Autodesk Fusion 360 part; units mm, degrees
(part 2 of 2)
sketch "Sketch49" plane through (0, 0, 3) normal (0, 0, 1) x (-1, 0, 0)
  line L0 (139.9, 32) -> (135, 32)
  line L1 (135, 32) -> (135, 34)
  line L2 (135, 34) -> (139.9, 34)
  line L3 (139.9, 34) -> (139.9, 32)
  circle A0 centre (127.45, 30.3) radius 1.5
  circle A1 centre (147.45, 30.3) radius 1.5
  arc A2 (127.45, 32.75) -> (127.45, 27.85) centre (127.45, 30.3) ccw
  line L4 (127.45, 27.85) -> (129.5, 27.85)
  line L5 (129.5, 27.85) -> (129.5, 25)
  line L6 (129.5, 25) -> (145.4, 25)
  line L7 (145.4, 25) -> (145.4, 27.85)
  line L8 (145.4, 27.85) -> (147.45, 27.85)
  arc A3 (147.45, 27.85) -> (147.45, 32.75) centre (147.45, 30.3) ccw
  line L9 (147.45, 32.75) -> (145.4, 32.75)
  line L10 (145.4, 32.75) -> (145.4, 35.6)
  line L11 (145.4, 35.6) -> (129.5, 35.6)
  line L12 (129.5, 35.6) -> (129.5, 32.75)
  line L13 (129.5, 32.75) -> (127.45, 32.75)
  line L14 (130, 25.5) -> (145, 25.5)
  line L15 (145, 25.5) -> (145, 27.5)
  line L16 (145, 27.5) -> (130, 27.5)
  line L17 (130, 27.5) -> (130, 25.5)
  constraint horizontal L14
  constraint vertical L15
  constraint horizontal L16
  constraint vertical L17
extrude "Extrude59" cut sketch "Sketch49" against normal blind 1 contours L14 L15 L16 L17 bodies 7
sketch "Sketch50" plane through (0, 0, 3) normal (0, 0, 1) x (-1, 0, 0)
  circle A0 centre (106.91, 41.51) radius 0.83
  circle A1 centre (106.91, 26.27) radius 0.83
  circle A2 centre (66.27, 41.51) radius 0.83
  circle A3 centre (66.27, 26.27) radius 0.83
  line L0 (65, 39) -> (71, 39)
  line L1 (71, 39) -> (71, 29)
  line L2 (71, 29) -> (65, 29)
  line L3 (65, 29) -> (65, 25)
  line L4 (65, 25) -> (108.18, 25)
  line L5 (108.18, 25) -> (108.18, 42.78)
  line L6 (108.18, 42.78) -> (65, 42.78)
  line L7 (65, 42.78) -> (65, 39)
  line L8 (105, 28) -> (93, 28)
  line L9 (93, 28) -> (93, 40)
  line L10 (93, 40) -> (105, 40)
  line L11 (105, 40) -> (105, 28)
  line L12 (76.4925, 33.236) -> (76.4925, 33)
  line L13 (76.4925, 33) -> (75, 33)
  line L14 (75, 33) -> (75, 35)
  line L15 (75, 35) -> (76.4461, 35)
  line L16 (76.4461, 35) -> (76.4461, 34.764)
  line L17 (76.4461, 34.764) -> (75.2647, 34.764)
  line L18 (75.2647, 34.764) -> (75.2647, 34.1514)
  line L19 (75.2647, 34.1514) -> (76.3711, 34.1514)
  line L20 (76.3711, 34.1514) -> (76.3711, 33.9168)
  line L21 (76.3711, 33.9168) -> (75.2647, 33.9168)
  line L22 (75.2647, 33.9168) -> (75.2647, 33.236)
  line L23 (75.2647, 33.236) -> (76.4925, 33.236)
  spline S0 degree 3 poles (82.4529, 33.369) (82.4332, 33.3474) (82.3952, 33.3057) (82.3642, 33.2587) (82.3493, 33.236) knots 0 0 0 0 0.008766 0.016888 0.016888 0.016888 0.016888
  line L24 (82.3493, 33.236) -> (83.3302, 33.236)
  line L25 (83.3302, 33.236) -> (83.3302, 33)
  line L26 (83.3302, 33) -> (82.0082, 33)
  spline S1 degree 3 poles (82.0082, 33) (82.0087, 33.0292) (82.0097, 33.0875) (82.0278, 33.1429) (82.0368, 33.1705) knots 0 0 0 0 0.008716 0.017379 0.017379 0.017379 0.017379
  spline S2 degree 3 poles (82.0368, 33.1705) (82.057, 33.2163) (82.0991, 33.312) (82.1644, 33.3938) (82.1985, 33.4366) knots 0 0 0 0 0.014925 0.031247 0.031247 0.031247 0.031247
  spline S3 degree 3 poles (82.1985, 33.4366) (82.2429, 33.4845) (82.3431, 33.5927) (82.4566, 33.687) (82.5198, 33.7394) knots 0 0 0 0 0.019599 0.044195 0.044195 0.044195 0.044195
  spline S4 degree 3 poles (82.5198, 33.7394) (82.6137, 33.8164) (82.7719, 33.9461) (82.9059, 34.1003) (82.9604, 34.163) knots 0 0 0 0 0.036337 0.061217 0.061217 0.061217 0.061217
  spline S5 degree 3 poles (82.9604, 34.163) (82.9938, 34.2119) (83.0551, 34.3018) (83.0688, 34.4094) (83.075, 34.4584) knots 0 0 0 0 0.017457 0.032082 0.032082 0.032082 0.032082
  spline S6 degree 3 poles (83.075, 34.4584) (83.0707, 34.5051) (83.0621, 34.5983) (83.0011, 34.6693) (82.9707, 34.7046) knots 0 0 0 0 0.013706 0.027345 0.027345 0.027345 0.027345
  spline S7 degree 3 poles (82.9707, 34.7046) (82.9322, 34.7339) (82.8519, 34.7948) (82.751, 34.8015) (82.6985, 34.8049) knots 0 0 0 0 0.014181 0.029581 0.029581 0.029581 0.029581
  spline S8 degree 3 poles (82.6985, 34.8049) (82.6432, 34.8014) (82.5376, 34.7945) (82.4544, 34.7295) (82.4147, 34.6985) knots 0 0 0 0 0.016182 0.030941 0.030941 0.030941 0.030941
  spline S9 degree 3 poles (82.4147, 34.6985) (82.3837, 34.6579) (82.3174, 34.5712) (82.3106, 34.4619) (82.307, 34.4038) knots 0 0 0 0 0.015007 0.032013 0.032013 0.032013 0.032013
  line L27 (82.307, 34.4038) -> (82.0546, 34.4297)
  spline S10 degree 3 poles (82.0546, 34.4297) (82.0672, 34.5164) (82.0908, 34.6793) (82.199, 34.8025) (82.2497, 34.8602) knots 0 0 0 0 0.025635 0.048167 0.048167 0.048167 0.048167
  spline S11 degree 3 poles (82.2497, 34.8602) (82.3136, 34.9033) (82.4505, 34.9955) (82.6159, 35.0038) (82.704, 35.0082) knots 0 0 0 0 0.022714 0.048594 0.048594 0.048594 0.048594
  spline S12 degree 3 poles (82.704, 35.0082) (82.793, 35.0033) (82.9609, 34.9941) (83.0961, 34.8951) (83.1596, 34.8486) knots 0 0 0 0 0.026091 0.049213 0.049213 0.049213 0.049213
  spline S13 degree 3 poles (83.1596, 34.8486) (83.2086, 34.792) (83.307, 34.6782) (83.3206, 34.5283) (83.3274, 34.4529) knots 0 0 0 0 0.021858 0.043952 0.043952 0.043952 0.043952
  spline S14 degree 3 poles (83.3274, 34.4529) (83.3253, 34.4129) (83.3209, 34.3317) (83.2926, 34.2555) (83.2783, 34.2169) knots 0 0 0 0 0.011966 0.024231 0.024231 0.024231 0.024231
  spline S15 degree 3 poles (83.2783, 34.2169) (83.2579, 34.1763) (83.2137, 34.0882) (83.1498, 34.0132) (83.1153, 33.9727) knots 0 0 0 0 0.013577 0.029457 0.029457 0.029457 0.029457
  spline S16 degree 3 poles (83.1153, 33.9727) (83.0654, 33.9213) (82.9453, 33.7975) (82.8137, 33.686) (82.7367, 33.6207) knots 0 0 0 0 0.021476 0.051719 0.051719 0.051719 0.051719
  spline S17 degree 3 poles (82.7367, 33.6207) (82.6755, 33.5697) (82.5783, 33.4886) (82.4868, 33.4013) (82.4529, 33.369) knots 0 0 0 0 0.023909 0.03794 0.03794 0.03794 0.03794
  spline S18 degree 3 poles (81.1228, 32.9645) (81.0397, 32.9702) (80.8789, 32.9811) (80.7486, 33.0757) (80.6855, 33.1214) knots 0 0 0 0 0.024413 0.047298 0.047298 0.047298 0.047298
  spline S19 degree 3 poles (80.6855, 33.1214) (80.6337, 33.1783) (80.5281, 33.2944) (80.5009, 33.4491) (80.487, 33.528) knots 0 0 0 0 0.022603 0.04608 0.04608 0.04608 0.04608
  line L28 (80.487, 33.528) -> (80.7326, 33.5607)
  spline S20 degree 3 poles (80.7326, 33.5607) (80.7468, 33.4984) (80.7721, 33.3868) (80.8445, 33.2988) (80.8765, 33.2599) knots 0 0 0 0 0.018844 0.033755 0.033755 0.033755 0.033755
  spline S21 degree 3 poles (80.8765, 33.2599) (80.9127, 33.233) (80.9862, 33.1784) (81.0776, 33.1714) (81.1241, 33.1678) knots 0 0 0 0 0.01322 0.026904 0.026904 0.026904 0.026904
  spline S22 degree 3 poles (81.1241, 33.1678) (81.1795, 33.1727) (81.2896, 33.1824) (81.3746, 33.2528) (81.4168, 33.2879) knots 0 0 0 0 0.016258 0.032307 0.032307 0.032307 0.032307
  spline S23 degree 3 poles (81.4168, 33.2879) (81.4516, 33.3306) (81.5221, 33.4173) (81.5314, 33.5288) (81.5362, 33.5853) knots 0 0 0 0 0.016147 0.032721 0.032721 0.032721 0.032721
  spline S24 degree 3 poles (81.5362, 33.5853) (81.532, 33.6387) (81.5239, 33.7433) (81.4579, 33.8246) (81.4256, 33.8643) knots 0 0 0 0 0.015678 0.030648 0.030648 0.030648 0.030648
  spline S25 degree 3 poles (81.4256, 33.8643) (81.3856, 33.8963) (81.3035, 33.962) (81.1985, 33.97) (81.1446, 33.9741) knots 0 0 0 0 0.015013 0.030806 0.030806 0.030806 0.030806
  spline S26 degree 3 poles (81.1446, 33.9741) (81.1185, 33.9725) (81.0599, 33.969) (81.0029, 33.9547) (80.9714, 33.9468) knots 0 0 0 0 0.00784 0.017573 0.017573 0.017573 0.017573
  line L29 (80.9714, 33.9468) -> (80.9986, 34.1623)
  spline S27 degree 3 poles (80.9986, 34.1623) (81.006, 34.1616) (81.0192, 34.1601) (81.0324, 34.1598) (81.0382, 34.1596) knots 0 0 0 0 0.002226 0.003967 0.003967 0.003967 0.003967
  spline S28 degree 3 poles (81.0382, 34.1596) (81.0889, 34.1629) (81.1892, 34.1693) (81.2771, 34.2176) (81.3206, 34.2415) knots 0 0 0 0 0.015044 0.029725 0.029725 0.029725 0.029725
  spline S29 degree 3 poles (81.3206, 34.2415) (81.3572, 34.2735) (81.4333, 34.3401) (81.4417, 34.4413) (81.4461, 34.4939) knots 0 0 0 0 0.014029 0.029194 0.029194 0.029194 0.029194
  spline S30 degree 3 poles (81.4461, 34.4939) (81.4426, 34.5367) (81.4356, 34.621) (81.3814, 34.6857) (81.3547, 34.7176) knots 0 0 0 0 0.012556 0.024703 0.024703 0.024703 0.024703
  spline S31 degree 3 poles (81.3547, 34.7176) (81.3212, 34.7435) (81.2518, 34.7971) (81.1641, 34.8031) (81.1187, 34.8063) knots 0 0 0 0 0.012404 0.025721 0.025721 0.025721 0.025721
  spline S32 degree 3 poles (81.1187, 34.8063) (81.0733, 34.8029) (80.9848, 34.7963) (80.9143, 34.7425) (80.8799, 34.7162) knots 0 0 0 0 0.013323 0.026012 0.026012 0.026012 0.026012
  spline S33 degree 3 poles (80.8799, 34.7162) (80.8507, 34.6802) (80.7864, 34.6012) (80.7675, 34.5007) (80.7572, 34.4461) knots 0 0 0 0 0.013719 0.030088 0.030088 0.030088 0.030088
  line L30 (80.7572, 34.4461) -> (80.5116, 34.4898)
  spline S34 degree 3 poles (80.5116, 34.4898) (80.53, 34.5662) (80.565, 34.7119) (80.6675, 34.8207) (80.7162, 34.8724) knots 0 0 0 0 0.023119 0.04407 0.04407 0.04407 0.04407
  spline S35 degree 3 poles (80.7162, 34.8724) (80.774, 34.912) (80.8935, 34.994) (81.0383, 35.0033) (81.1132, 35.0082) knots 0 0 0 0 0.020598 0.042654 0.042654 0.042654 0.042654
  spline S36 degree 3 poles (81.1132, 35.0082) (81.1664, 35.0054) (81.2711, 35) (81.3673, 34.9584) (81.4147, 34.9379) knots 0 0 0 0 0.015821 0.03118 0.03118 0.03118 0.03118
  spline S37 degree 3 poles (81.4147, 34.9379) (81.4577, 34.9129) (81.5416, 34.8639) (81.598, 34.7848) (81.6255, 34.7462) knots 0 0 0 0 0.014725 0.02878 0.02878 0.02878 0.02878
  spline S38 degree 3 poles (81.6255, 34.7462) (81.6468, 34.7054) (81.689, 34.6245) (81.6953, 34.5335) (81.6985, 34.4884) knots 0 0 0 0 0.013662 0.027054 0.027054 0.027054 0.027054
  spline S39 degree 3 poles (81.6985, 34.4884) (81.6957, 34.4463) (81.69, 34.3624) (81.6492, 34.2889) (81.6289, 34.2524) knots 0 0 0 0 0.012502 0.024877 0.024877 0.024877 0.024877
  spline S40 degree 3 poles (81.6289, 34.2524) (81.602, 34.2183) (81.5457, 34.147) (81.465, 34.1051) (81.4229, 34.0832) knots 0 0 0 0 0.012871 0.026927 0.026927 0.026927 0.026927
  spline S41 degree 3 poles (81.4229, 34.0832) (81.4782, 34.0666) (81.5853, 34.0345) (81.6616, 33.9529) (81.6985, 33.9134) knots 0 0 0 0 0.016967 0.032892 0.032892 0.032892 0.032892
  spline S42 degree 3 poles (81.6985, 33.9134) (81.7271, 33.8663) (81.7873, 33.7673) (81.7935, 33.6514) (81.7967, 33.5907) knots 0 0 0 0 0.016275 0.034196 0.034196 0.034196 0.034196
  spline S43 degree 3 poles (81.7967, 33.5907) (81.7887, 33.5067) (81.7726, 33.3382) (81.6614, 33.2106) (81.6057, 33.1467) knots 0 0 0 0 0.024665 0.049435 0.049435 0.049435 0.049435
  spline S44 degree 3 poles (81.6057, 33.1467) (81.5366, 33.0935) (81.3942, 32.9843) (81.2149, 32.9712) (81.1228, 32.9645) knots 0 0 0 0 0.025577 0.052634 0.052634 0.052634 0.052634
  line L31 (78.9864, 33.8131) -> (78.9864, 33)
  line L32 (78.9864, 33) -> (78.7217, 33)
  line L33 (78.7217, 33) -> (78.7217, 35)
  line L34 (78.7217, 35) -> (79.4761, 35)
  spline S45 degree 3 poles (79.4761, 35) (79.5348, 34.9998) (79.6366, 34.9995) (79.7375, 34.9864) (79.7804, 34.9809) knots 0 0 0 0 0.017571 0.030509 0.030509 0.030509 0.030509
  spline S46 degree 3 poles (79.7804, 34.9809) (79.8265, 34.9715) (79.9139, 34.9538) (79.9909, 34.9088) (80.0273, 34.8874) knots 0 0 0 0 0.014001 0.026563 0.026563 0.026563 0.026563
  spline S47 degree 3 poles (80.0273, 34.8874) (80.0592, 34.8615) (80.1253, 34.8078) (80.1663, 34.7331) (80.1876, 34.6944) knots 0 0 0 0 0.012214 0.025303 0.025303 0.025303 0.025303
  spline S48 degree 3 poles (80.1876, 34.6944) (80.2053, 34.6515) (80.2414, 34.5642) (80.246, 34.4697) (80.2483, 34.4216) knots 0 0 0 0 0.013801 0.028138 0.028138 0.028138 0.028138
  spline S49 degree 3 poles (80.2483, 34.4216) (80.242, 34.3403) (80.2296, 34.1805) (80.1333, 34.0526) (80.0859, 33.9898) knots 0 0 0 0 0.023898 0.046996 0.046996 0.046996 0.046996
  spline S50 degree 3 poles (80.0859, 33.9898) (80.0124, 33.9386) (79.8379, 33.8171) (79.6234, 33.8146) (79.4993, 33.8131) knots 0 0 0 0 0.026356 0.062507 0.062507 0.062507 0.062507
  line L35 (79.4993, 33.8131) -> (78.9864, 33.8131)
  spline S51 degree 3 poles (77.1658, 33.045) (77.1081, 33.0744) (76.9944, 33.1323) (76.9164, 33.2333) (76.8779, 33.2831) knots 0 0 0 0 0.019136 0.037772 0.037772 0.037772 0.037772
  spline S52 degree 3 poles (76.8779, 33.2831) (76.8472, 33.3383) (76.785, 33.4502) (76.7738, 33.5778) (76.7681, 33.6426) knots 0 0 0 0 0.018713 0.037965 0.037965 0.037965 0.037965
  line L36 (76.7681, 33.6426) -> (77.0177, 33.6644)
  spline S53 degree 3 poles (77.0177, 33.6644) (77.0248, 33.6179) (77.038, 33.5309) (77.0805, 33.454) (77.1003, 33.4181) knots 0 0 0 0 0.013975 0.026155 0.026155 0.026155 0.026155
  spline S54 degree 3 poles (77.1003, 33.4181) (77.1262, 33.3871) (77.1817, 33.3205) (77.2598, 33.2827) (77.3015, 33.2626) knots 0 0 0 0 0.012002 0.025694 0.025694 0.025694 0.025694
  spline S55 degree 3 poles (77.3015, 33.2626) (77.3493, 33.2453) (77.4485, 33.2094) (77.5539, 33.2054) (77.6085, 33.2033) knots 0 0 0 0 0.015163 0.031432 0.031432 0.031432 0.031432
  spline S56 degree 3 poles (77.6085, 33.2033) (77.6564, 33.2047) (77.7476, 33.2075) (77.8346, 33.2352) (77.8759, 33.2483) knots 0 0 0 0 0.014301 0.027232 0.027232 0.027232 0.027232
  spline S57 degree 3 poles (77.8759, 33.2483) (77.9113, 33.2637) (77.9778, 33.2926) (78.0259, 33.3466) (78.0484, 33.3718) knots 0 0 0 0 0.011435 0.021444 0.021444 0.021444 0.021444
  spline S58 degree 3 poles (78.0484, 33.3718) (78.0649, 33.3983) (78.0976, 33.4509) (78.1026, 33.5125) (78.105, 33.543) knots 0 0 0 0 0.009237 0.018267 0.018267 0.018267 0.018267
  spline S59 degree 3 poles (78.105, 33.543) (78.1029, 33.5732) (78.0987, 33.6327) (78.0664, 33.6827) (78.0505, 33.7074) knots 0 0 0 0 0.008921 0.017573 0.017573 0.017573 0.017573
  spline S60 degree 3 poles (78.0505, 33.7074) (78.0275, 33.7305) (77.9759, 33.7824) (77.908, 33.8101) (77.8704, 33.8254) knots 0 0 0 0 0.009698 0.021725 0.021725 0.021725 0.021725
  spline S61 degree 3 poles (77.8704, 33.8254) (77.8274, 33.8392) (77.7102, 33.8767) (77.5903, 33.905) (77.5143, 33.9229) knots 0 0 0 0 0.013533 0.036931 0.036931 0.036931 0.036931
  spline S62 degree 3 poles (77.5143, 33.9229) (77.4354, 33.9418) (77.3033, 33.9733) (77.1784, 34.0264) (77.1282, 34.0477) knots 0 0 0 0 0.024297 0.040637 0.040637 0.040637 0.040637
  spline S63 degree 3 poles (77.1282, 34.0477) (77.0843, 34.0732) (77.0008, 34.1214) (76.9424, 34.1978) (76.9147, 34.234) knots 0 0 0 0 0.015064 0.02858 0.02858 0.02858 0.02858
  spline S64 degree 3 poles (76.9147, 34.234) (76.8942, 34.2724) (76.8527, 34.3503) (76.8473, 34.4384) (76.8445, 34.4829) knots 0 0 0 0 0.012908 0.026139 0.026139 0.026139 0.026139
  spline S65 degree 3 poles (76.8445, 34.4829) (76.8482, 34.5328) (76.8557, 34.6336) (76.9054, 34.7216) (76.9304, 34.766) knots 0 0 0 0 0.014805 0.02991 0.02991 0.02991 0.02991
  spline S66 degree 3 poles (76.9304, 34.766) (76.9633, 34.8076) (77.0312, 34.8938) (77.1302, 34.9413) (77.1814, 34.9659) knots 0 0 0 0 0.01568 0.032466 0.032466 0.032466 0.032466
  spline S67 degree 3 poles (77.1814, 34.9659) (77.239, 34.9858) (77.3579, 35.0269) (77.4836, 35.0316) (77.5484, 35.0341) knots 0 0 0 0 0.018164 0.037509 0.037509 0.037509 0.037509
  spline S68 degree 3 poles (77.5484, 35.0341) (77.6189, 35.0317) (77.7532, 35.0272) (77.8802, 34.9834) (77.9407, 34.9625) knots 0 0 0 0 0.021001 0.040071 0.040071 0.040071 0.040071
  spline S69 degree 3 poles (77.9407, 34.9625) (77.9936, 34.9365) (78.0966, 34.8858) (78.1674, 34.7956) (78.2019, 34.7517) knots 0 0 0 0 0.017437 0.033952 0.033952 0.033952 0.033952
  spline S70 degree 3 poles (78.2019, 34.7517) (78.2289, 34.7034) (78.2836, 34.6052) (78.2946, 34.4933) (78.3001, 34.4366) knots 0 0 0 0 0.016416 0.033327 0.033327 0.033327 0.033327
  line L37 (78.3001, 34.4366) -> (78.0464, 34.4175)
  spline S71 degree 3 poles (78.0464, 34.4175) (78.0368, 34.4756) (78.0189, 34.5852) (77.9433, 34.666) (77.9079, 34.704) knots 0 0 0 0 0.017238 0.032462 0.032462 0.032462 0.032462
  spline S72 degree 3 poles (77.9079, 34.704) (77.8604, 34.7321) (77.7535, 34.7955) (77.6287, 34.7989) (77.5593, 34.8008) knots 0 0 0 0 0.016321 0.036707 0.036707 0.036707 0.036707
  spline S73 degree 3 poles (77.5593, 34.8008) (77.4884, 34.7997) (77.3642, 34.7979) (77.2559, 34.7384) (77.2094, 34.7128) knots 0 0 0 0 0.02087 0.036564 0.036564 0.036564 0.036564
  spline S74 degree 3 poles (77.2094, 34.7128) (77.1774, 34.6828) (77.1156, 34.6248) (77.1048, 34.5411) (77.0996, 34.5007) knots 0 0 0 0 0.012728 0.024562 0.024562 0.024562 0.024562
  spline S75 degree 3 poles (77.0996, 34.5007) (77.1027, 34.4665) (77.1089, 34.3986) (77.1547, 34.3483) (77.1774, 34.3233) knots 0 0 0 0 0.010013 0.019843 0.019843 0.019843 0.019843
  spline S76 degree 3 poles (77.1774, 34.3233) (77.2227, 34.2981) (77.3472, 34.2287) (77.4873, 34.1994) (77.5764, 34.1808) knots 0 0 0 0 0.01549 0.042576 0.042576 0.042576 0.042576
  spline S77 degree 3 poles (77.5764, 34.1808) (77.6678, 34.1603) (77.818, 34.1268) (77.9625, 34.0739) (78.0191, 34.0532) knots 0 0 0 0 0.028046 0.046113 0.046113 0.046113 0.046113
  spline S78 degree 3 poles (78.0191, 34.0532) (78.0724, 34.0262) (78.1723, 33.9754) (78.2437, 33.8894) (78.2769, 33.8493) knots 0 0 0 0 0.017708 0.033187 0.033187 0.033187 0.033187
  spline S79 degree 3 poles (78.2769, 33.8493) (78.3012, 33.806) (78.3508, 33.7176) (78.357, 33.6165) (78.3602, 33.5648) knots 0 0 0 0 0.014678 0.02998 0.02998 0.02998 0.02998
  spline S80 degree 3 poles (78.3602, 33.5648) (78.3561, 33.512) (78.348, 33.405) (78.2954, 33.3114) (78.2688, 33.264) knots 0 0 0 0 0.015669 0.031781 0.031781 0.031781 0.031781
  spline S81 degree 3 poles (78.2688, 33.264) (78.2342, 33.2192) (78.1628, 33.1268) (78.0594, 33.0724) (78.0061, 33.0443) knots 0 0 0 0 0.016779 0.034595 0.034595 0.034595 0.034595
  spline S82 degree 3 poles (78.0061, 33.0443) (77.9462, 33.0215) (77.8221, 32.9741) (77.6893, 32.9687) (77.6207, 32.9659) knots 0 0 0 0 0.019123 0.039562 0.039562 0.039562 0.039562
  spline S83 degree 3 poles (77.6207, 32.9659) (77.5368, 32.968) (77.381, 32.972) (77.2337, 33.022) (77.1658, 33.045) knots 0 0 0 0 0.025027 0.046416 0.046416 0.046416 0.046416
  line L38 (68, 25) -> (105, 25)
  line L39 (105, 25) -> (105, 27)
  line L40 (105, 27) -> (68, 27)
  line L41 (68, 27) -> (68, 25)
  line L42 (68, 41) -> (68, 42.78)
  line L43 (68, 42.78) -> (105, 42.78)
  line L44 (105, 42.78) -> (105, 40.78)
  line L45 (105, 40.78) -> (68, 40.78)
  line L46 (68, 40.78) -> (68, 42.78)
  dimension "d258" = 2
  constraint horizontal L38
  constraint vertical L39
  constraint horizontal L40
  constraint vertical L41
  constraint coincident L4 L38.start
  constraint coincident L6 L42.end
  constraint perpendicular L6 L42
  constraint horizontal L43
  constraint vertical L44
  constraint horizontal L45
  constraint vertical L46
  measures "d258" distance of L42.end L45.end
extrude "Extrude60" cut sketch "Sketch50" against normal blind 1 contours L6 L42 L43 L44 L45 L46 | L4 L38 L39 L40 L41 bodies 4
sketch "Sketch51" plane through (0, 0, 2) normal (0, 0, 1) x (-1, 0, 0)
  line L0 (68, 27) -> (68, 25)
  line L1 (68, 25) -> (105, 25)
  line L2 (105, 25) -> (105, 27)
  line L3 (105, 27) -> (68, 27)
sketch "Sketch52" plane through (0, 0, 3) normal (0, 0, 1) x (-1, 0, 0)
  line L0 (145, 25.5) -> (130, 25.5)
  line L1 (130, 25.5) -> (130, 27.5)
  line L2 (130, 27.5) -> (145, 27.5)
  line L3 (145, 27.5) -> (145, 25.5)
  line L4 (139.9, 32) -> (135, 32)
  line L5 (135, 32) -> (135, 34)
  line L6 (135, 34) -> (139.9, 34)
  line L7 (139.9, 34) -> (139.9, 32)
  circle A0 centre (127.45, 30.3) radius 1.5
  circle A1 centre (147.45, 30.3) radius 1.5
  arc A2 (127.45, 32.75) -> (127.45, 27.85) centre (127.45, 30.3) ccw
  line L8 (127.45, 27.85) -> (129.5, 27.85)
  line L9 (129.5, 27.85) -> (129.5, 25)
  line L10 (129.5, 25) -> (145.4, 25)
  line L11 (145.4, 25) -> (145.4, 27.85)
  line L12 (145.4, 27.85) -> (147.45, 27.85)
  arc A3 (147.45, 27.85) -> (147.45, 32.75) centre (147.45, 30.3) ccw
  line L13 (147.45, 32.75) -> (145.4, 32.75)
  line L14 (145.4, 32.75) -> (145.4, 35.6)
  line L15 (145.4, 35.6) -> (129.5, 35.6)
  line L16 (129.5, 35.6) -> (129.5, 32.75)
  line L17 (129.5, 32.75) -> (127.45, 32.75)
  line L18 (135.0059, 30.3197) -> (139.9059, 30.3369) construction
  line L19 (139.9059, 30.3369) -> (139.9, 32.0172) construction
  line L20 (139.9, 32.0172) -> (135, 32) construction
  line L21 (135, 32) -> (135.0059, 30.3197) construction
  dimension "d265" = 2
  text T0 "ToF" font "Arial" height 2 align centre top in box 4.9 x 1.6803 at (135.0059, 30.3197) x (0.999994, 0.003504) y (-0.003504, 0.999994) spacing 1 kerned
  constraint coincident L4.end
extrude "Extrude61" cut sketch "Sketch52" against normal blind 1 text T0 bodies 7
copy_body "CopyPasteBodies1" bodies 7 makes body 8
move_body "Move2" bodies 8 to x (1, 0, 0) y (0, 1, 0) z (0, 0, 1) at (0.0526, -14.9999, 0)
sketch "Sketch53" plane through (0, 0, 0) normal (0, 0, 1) x (1, 0, 0)
  line L0 (0, -95) -> (-20, -95)
  line L1 (-20, -95) -> (-20, -112.8)
  line L2 (-20, -112.8) -> (0, -112.8)
  line L3 (0, -112.8) -> (0, -95)
  line L4 (-20, -112.8) -> (-7, -112.8)
  line L5 (-7, -112.8) -> (-7, -117.5)
  line L6 (-7, -117.5) -> (-20, -117.5)
  line L7 (-20, -117.5) -> (-20, -112.8)
  line L8 (0, -110) -> (3.8, -110)
  line L9 (3.8, -110) -> (3.8, -109)
  line L10 (3.8, -109) -> (0, -109)
  line L11 (0, -109) -> (0, -110)
  line L12 (-20, -110) -> (-23.8, -110)
  line L13 (-23.8, -110) -> (-23.8, -109)
  line L14 (-23.8, -109) -> (-20, -109)
  line L15 (-20, -109) -> (-20, -110)
  dimension "d269" = 20
  dimension "d270" = 17.8
  dimension "d271" = 4.7
  dimension "d272" = 3.8
  dimension "d273" = 1
  dimension "d274" = 3.8
  constraint horizontal L0
  constraint vertical L1
  constraint horizontal L2
  constraint vertical L3
  constraint horizontal L4
  constraint vertical L5
  constraint horizontal L6
  constraint vertical L7
  constraint horizontal L8
  constraint vertical L9
  constraint horizontal L10
  constraint vertical L11
  constraint coincident L3 L8.start
  constraint horizontal L12
  constraint vertical L13
  constraint horizontal L14
  constraint vertical L15
  constraint coincident L1 L12.start
  measures "d269" distance of L0.start L0.end
  measures "d270" distance of L0.start L2.end
  measures "d271" distance of L1.end L6.end
  measures "d272" distance of L8.start L8.end
  measures "d273" distance of L8.start L10.end
  measures "d274" distance of L12.start L12.end
extrude "Extrude62" add sketch "Sketch53" along normal blind 8 separate body makes body 9
sketch "Sketch54" plane through (0, -117.5, 0) normal (0, -1, 0) x (1, 0, 0)
  line L0 (-20, 0) -> (-7, 0)
  line L1 (-7, 0) -> (-7, 8)
  line L2 (-7, 8) -> (-20, 8)
  line L3 (-20, 8) -> (-20, 0)
  circle A0 centre (-16, 4) radius 3.75
  dimension "d277" = 7.5
  measures "d277" diameter of A0
extrude "Extrude63" cut sketch "Sketch54" against normal blind 2 bodies 9
sketch "Sketch55" plane through (0, -115.5, 0) normal (0, -1, 0) x (1, 0, 0)
  circle A0 centre (-16, 4) radius 3.75
  line L0 (-20, 8) -> (-20, 0)
  line L1 (-20, 0) -> (-7, 0)
  line L2 (-7, 0) -> (-7, 8)
  line L3 (-7, 8) -> (-20, 8)
  line L4 (-16, 8) -> (-7.7253, 5.6358)
  line L5 (-16, 0) -> (-7.7253, 2.3642)
  line L6 (-7, 3.3257) -> (-7, 4.6743)
  arc A1 (-7.7253, 2.3642) -> (-7, 3.3257) centre (-8, 3.3257) ccw
  arc A2 (-7, 4.6743) -> (-7.7253, 5.6358) centre (-8, 4.6743) ccw
  dimension "d280" = 1
  constraint coincident L3 L4.start
  constraint coincident L1 L5.start
  constraint tangent L6 A1
  constraint tangent L5 A1
  constraint tangent L4 A2
  constraint tangent L6 A2
  constraint equal A1 A2
  measures "d280" radius of A1
extrude "Extrude64" cut sketch "Sketch55" against normal blind 2.7 contours L2 L3 L4 A2 | L1 L2 L5 A1 bodies 9
extrude "Extrude65" add 1 faces at (-128, 20.0864, 4.8227) along direction (-1, 0, 0) blind 1 on bodies 6 bodies 6
sketch "Sketch56" plane through (0, 0, 0) normal (0, 0, 1) x (1, 0, 0)
  line L0 (-35, -95) -> (-52.1, -95)
  line L1 (-52.1, -95) -> (-52.1, -116.6)
  line L2 (-52.1, -116.6) -> (-35, -116.6)
  line L3 (-35, -116.6) -> (-35, -95)
  dimension "d285" = 17.1
  dimension "d286" = 21.6
  constraint horizontal L0
  constraint vertical L1
  constraint horizontal L2
  constraint vertical L3
  measures "d285" distance of L0.start L0.end
  measures "d286" distance of L0.start L2.end
extrude "Extrude66" add sketch "Sketch56" along normal blind 3 separate body makes body 10
sketch "Sketch57" plane through (0, 0, 3) normal (0, 0, 1) x (-1, 0, 0)
  line L0 (35, 116.6) -> (35, 95)
  line L1 (35, 95) -> (52.1, 95)
  line L2 (52.1, 95) -> (52.1, 116.6)
  line L3 (52.1, 116.6) -> (35, 116.6)
  circle A0 centre (49.5, 114) radius 2
  dimension "d289" = 4
  measures "d289" diameter of A0
extrude "Extrude67" cut sketch "Sketch57" against normal blind 4.5 contours A0 bodies 10
sketch "Sketch58" plane through (0, 0, 3) normal (0, 0, 1) x (-1, 0, 0)
  circle A0 centre (49.5, 114) radius 2
  line L0 (35, 116.6) -> (35, 95)
  line L1 (35, 95) -> (52.1, 95)
  line L2 (52.1, 95) -> (52.1, 116.6)
  line L3 (52.1, 116.6) -> (35, 116.6)
  line L4 (37, 116) -> (35, 116)
  line L5 (35, 116) -> (35, 96)
  line L6 (35, 96) -> (37, 96)
  line L7 (37, 96) -> (37, 116)
  constraint horizontal L4
  constraint vertical L5
  constraint horizontal L6
  constraint vertical L7
  constraint coincident L0 L5.end
extrude "Extrude68" cut sketch "Sketch58" against normal blind 1 contours L0 L4 L5 L6 L7 bodies 10
sketch "Sketch59" plane through (0, 0, 3) normal (0, 0, 1) x (-1, 0, 0)
  line L0 (37, 96) -> (35, 96)
  line L1 (35, 96) -> (35, 95)
  line L2 (35, 95) -> (52.1, 95)
  line L3 (52.1, 95) -> (52.1, 116.6)
  line L4 (52.1, 116.6) -> (35, 116.6)
  line L5 (35, 116.6) -> (35, 116)
  line L6 (35, 116) -> (37, 116)
  line L7 (37, 116) -> (37, 96)
  circle A0 centre (49.5, 114) radius 2
  line L8 (45, 110) -> (48, 110)
  line L9 (48, 110) -> (48, 107)
  line L10 (48, 107) -> (45, 107)
  line L11 (45, 107) -> (45, 110)
  line L12 (45, 105) -> (47, 105)
  line L13 (47, 105) -> (47, 103)
  line L14 (47, 103) -> (45, 103)
  line L15 (45, 103) -> (45, 105)
  line L16 (39, 113) -> (41, 113)
  line L17 (41, 113) -> (41, 112)
  line L18 (41, 112) -> (39, 112)
  line L19 (39, 112) -> (39, 113)
  constraint horizontal L8
  constraint vertical L9
  constraint horizontal L10
  constraint vertical L11
  constraint horizontal L12
  constraint vertical L13
  constraint horizontal L14
  constraint vertical L15
  constraint horizontal L16
  constraint vertical L17
  constraint horizontal L18
  constraint vertical L19
extrude "Extrude69" add sketch "Sketch59" along normal blind 1 contours L8 L9 L10 L11 | L12 L13 L14 L15 | L16 L17 L18 L19 bodies 10
sketch "Sketch60" plane through (0, 0, 3) normal (0, 0, 1) x (-1, 0, 0)
  line L0 (45, 103) -> (45, 105)
  line L1 (45, 105) -> (47, 105)
  line L2 (47, 105) -> (47, 103)
  line L3 (47, 103) -> (45, 103)
  line L4 (45, 107) -> (45, 110)
  line L5 (45, 110) -> (48, 110)
  line L6 (48, 110) -> (48, 107)
  line L7 (48, 107) -> (45, 107)
  line L8 (39, 112) -> (39, 113)
  line L9 (39, 113) -> (41, 113)
  line L10 (41, 113) -> (41, 112)
  line L11 (41, 112) -> (39, 112)
  line L12 (37, 96) -> (35, 96)
  line L13 (35, 96) -> (35, 95)
  line L14 (35, 95) -> (52.1, 95)
  line L15 (52.1, 95) -> (52.1, 116.6)
  line L16 (52.1, 116.6) -> (35, 116.6)
  line L17 (35, 116.6) -> (35, 116)
  line L18 (35, 116) -> (37, 116)
  line L19 (37, 116) -> (37, 96)
  circle A0 centre (49.5, 114) radius 2
  line L20 (37, 97.7) -> (52.1, 97.7) construction
  line L21 (52.1, 97.7) -> (52.1, 101) construction
  line L22 (52.1, 101) -> (37, 101) construction
  line L23 (37, 101) -> (37, 97.7) construction
  dimension "d296" = 2
  text T0 "IMU" font "Arial" height 2 align centre top in box 15.1 x 3.3 at (37, 97.7) x (1, 0) y (0, 1) spacing 1 kerned
  constraint coincident L15
  constraint coincident L19
extrude "Extrude70" cut sketch "Sketch60" against normal blind 1 text T0 bodies 10
sketch "Sketch61" plane through (0, 0, 0) normal (0, 0, 1) x (1, 0, 0)
  line L0 (-70, -95) -> (-80, -95)
  line L1 (-80, -95) -> (-80, -113)
  line L2 (-80, -113) -> (-70, -113)
  line L3 (-70, -113) -> (-70, -95)
  dimension "d300" = 10
  dimension "d301" = 18
  constraint horizontal L0
  constraint vertical L1
  constraint horizontal L2
  constraint vertical L3
  measures "d300" distance of L0.start L0.end
  measures "d301" distance of L0.start L2.end
extrude "Extrude71" add sketch "Sketch61" along normal blind 3 separate body makes body 11
sketch "Sketch62" plane through (0, 0, 3) normal (0, 0, 1) x (-1, 0, 0)
  line L0 (70, 113) -> (70, 95)
  line L1 (70, 95) -> (80, 95)
  line L2 (80, 95) -> (80, 113)
  line L3 (80, 113) -> (70, 113)
  line L4 (71, 113) -> (79, 113)
  line L5 (79, 113) -> (79, 111)
  line L6 (79, 111) -> (71, 111)
  line L7 (71, 111) -> (71, 113)
  circle A0 centre (73, 98) radius 2.2361
  line L8 (76, 101) -> (79, 101)
  line L9 (79, 101) -> (79, 97)
  line L10 (79, 97) -> (76, 97)
  line L11 (76, 97) -> (76, 101)
  constraint horizontal L4
  constraint vertical L5
  constraint horizontal L6
  constraint vertical L7
  constraint coincident L3 L4.start
  constraint horizontal L8
  constraint vertical L9
  constraint horizontal L10
  constraint vertical L11
extrude "Extrude72" add sketch "Sketch62" along normal blind 2 contours L3 L4 L5 L6 L7 | A0 | L8 L9 L10 L11 bodies 11
sketch "Sketch63" plane through (0, -113, 0) normal (0, -1, 0) x (1, 0, 0)
  line L0 (-80, 0) -> (-70, 0)
  line L1 (-70, 0) -> (-70, 3)
  line L2 (-70, 3) -> (-71, 3)
  line L3 (-71, 3) -> (-71, 5)
  line L4 (-71, 5) -> (-79, 5)
  line L5 (-79, 5) -> (-79, 3)
  line L6 (-79, 3) -> (-80, 3)
  line L7 (-80, 3) -> (-80, 0)
  circle A0 centre (-77.5, 4) radius 0.5385
  circle A1 centre (-72.5, 4) radius 0.5099
  circle A2 centre (-75, 4) radius 0.5
extrude "Extrude73" add sketch "Sketch63" along normal blind 6 contours A0 | A1 | A2 bodies 11
sketch "Sketch64" plane through (0, 0, 3) normal (0, 0, 1) x (-1, 0, 0)
  line L0 (76, 97) -> (76, 101)
  line L1 (76, 101) -> (79, 101)
  line L2 (79, 101) -> (79, 97)
  line L3 (79, 97) -> (76, 97)
  circle A0 centre (73, 98) radius 2.2361
  line L4 (79, 113) -> (79, 111)
  line L5 (79, 111) -> (71, 111)
  line L6 (71, 111) -> (71, 113)
  line L7 (71, 113) -> (70, 113)
  line L8 (70, 113) -> (70, 95)
  line L9 (70, 95) -> (80, 95)
  line L10 (80, 95) -> (80, 113)
  line L11 (80, 113) -> (79, 113)
  line L12 (71, 108) -> (79, 108) construction
  line L13 (79, 108) -> (79, 110) construction
  line L14 (79, 110) -> (71, 110) construction
  line L15 (71, 110) -> (71, 108) construction
  line L16 (71, 102) -> (79, 102) construction
  line L17 (79, 102) -> (79, 104) construction
  line L18 (79, 104) -> (71, 104) construction
  line L19 (71, 104) -> (71, 102) construction
  dimension "d308" = 2
  dimension "d310" = 2
  dimension "d311" = 0
  text T0 "Step Down" font "Arial" height 2 align centre top in box 8 x 2 at (71, 108) x (1, 0) y (0, 1) spacing 1 kerned
  text T1 "(5V)" font "Arial" height 2 align centre top in box 8 x 2 at (71, 102) x (1, 0) y (0, 1) spacing 1 kerned
extrude "Extrude74" cut sketch "Sketch64" against normal blind 1 text T0 T1 bodies 11
sketch "Sketch65" plane through (0, 0, 0) normal (0, 0, 1) x (1, 0, 0)
  line L0 (-110, -95) -> (-146, -95)
  line L1 (-146, -95) -> (-146, -166)
  line L2 (-146, -166) -> (-110, -166)
  line L3 (-110, -166) -> (-110, -95)
  dimension "d314" = 36
  dimension "d315" = 71
  constraint horizontal L0
  constraint vertical L1
  constraint horizontal L2
  constraint vertical L3
  measures "d314" distance of L0.start L0.end
  measures "d315" distance of L0.start L2.end
extrude "Extrude75" add sketch "Sketch65" along normal blind 20 separate body makes body 12
sketch "Sketch66" plane through (0, -166, 0) normal (0, -1, 0) x (1, 0, 0)
  line L0 (-146, 0) -> (-110, 0)
  line L1 (-110, 0) -> (-110, 20)
  line L2 (-110, 20) -> (-146, 20)
  line L3 (-146, 20) -> (-146, 0)
  circle A0 centre (-141, 15) radius 4.1231
extrude "Extrude76" add sketch "Sketch66" along normal blind 10 contours A0 bodies 12
sketch "Sketch67" plane through (0, 0, 20) normal (0, 0, 1) x (-1, 0, 0)
  line L0 (110, 166) -> (110, 95)
  line L1 (110, 95) -> (146, 95)
  line L2 (146, 95) -> (146, 166)
  line L3 (146, 166) -> (110, 166)
  line L4 (115, 155) -> (140, 155) construction
  line L5 (140, 155) -> (140, 160) construction
  line L6 (140, 160) -> (115, 160) construction
  line L7 (115, 160) -> (115, 155) construction
  dimension "d320" = 4
  text T0 "LiPo Battery" font "Arial" height 4 align centre top in box 25 x 5 at (115, 155) x (1, 0) y (0, 1) spacing 1 kerned
extrude "Extrude77" cut sketch "Sketch67" against normal blind 1 text T0 bodies 12
sketch "Sketch68" plane through (0, 0, 0) normal (0, 0, 1) x (1, 0, 0)
  line L0 (0, -125) -> (-10.16, -125)
  line L1 (-10.16, -125) -> (-10.16, -145.5)
  line L2 (-10.16, -145.5) -> (0, -145.5)
  line L3 (0, -145.5) -> (0, -125)
  dimension "d324" = 10.16
  dimension "d325" = 20.5
  constraint horizontal L0
  constraint vertical L1
  constraint horizontal L2
  constraint vertical L3
  measures "d324" distance of L0.start L0.end
  measures "d325" distance of L0.start L2.end
extrude "Extrude78" add sketch "Sketch68" along normal blind 3 separate body makes body 13
sketch "Sketch69" plane through (0, 0, 3) normal (0, 0, 1) x (-1, 0, 0)
  line L0 (0, 145.5) -> (0, 125)
  line L1 (0, 125) -> (10.16, 125)
  line L2 (10.16, 125) -> (10.16, 145.5)
  line L3 (10.16, 145.5) -> (0, 145.5)
  circle A0 centre (7, 142.5) radius 2.5495
  line L4 (1, 144) -> (3.5, 144)
  line L5 (3.5, 144) -> (3.5, 139)
  line L6 (3.5, 139) -> (1, 139)
  line L7 (1, 139) -> (1, 144)
  line L8 (5, 139.5) -> (7.5, 139.5)
  line L9 (7.5, 139.5) -> (7.5, 137)
  line L10 (7.5, 137) -> (5, 137)
  line L11 (5, 137) -> (5, 139.5)
  line L12 (8.5, 139) -> (9.5, 139)
  line L13 (9.5, 139) -> (9.5, 137.5)
  line L14 (9.5, 137.5) -> (8.5, 137.5)
  line L15 (8.5, 137.5) -> (8.5, 139)
  line L16 (0.5, 127.5) -> (9.5, 127.5)
  line L17 (9.5, 127.5) -> (9.5, 125)
  line L18 (9.5, 125) -> (0.5, 125)
  line L19 (0.5, 125) -> (0.5, 127.5)
  constraint horizontal L4
  constraint vertical L5
  constraint horizontal L6
  constraint vertical L7
  constraint horizontal L8
  constraint vertical L9
  constraint horizontal L10
  constraint vertical L11
  constraint horizontal L12
  constraint vertical L13
  constraint horizontal L14
  constraint vertical L15
  constraint horizontal L16
  constraint vertical L17
  constraint horizontal L18
  constraint vertical L19
extrude "Extrude79" add sketch "Sketch69" along normal blind 2 contours L1 L16 L17 L18 L19 | A0 | L4 L5 L6 L7 | L8 L9 L10 L11 | L12 L13 L14 L15 bodies 13
extrude "Extrude80" add 1 faces at (-3.5, -126.6667, 5) along direction (0, 0, 1) blind 0.6 on bodies 13 bodies 13
sketch "Sketch70" plane through (0, -125, 0) normal (0, 1, 0) x (-1, 0, 0)
  line L0 (0, 0) -> (10.16, 0)
  line L1 (10.16, 0) -> (10.16, 3)
  line L2 (10.16, 3) -> (9.5, 3)
  line L3 (9.5, 3) -> (9.5, 5.6)
  line L4 (9.5, 5.6) -> (0.5, 5.6)
  line L5 (0.5, 5.6) -> (0.5, 3)
  line L6 (0.5, 3) -> (0, 3)
  line L7 (0, 3) -> (0, 0)
  circle A0 centre (1.6166, 4.3) radius 0.5
  circle A1 centre (3.5103, 4.3) radius 0.5
  circle A2 centre (5.5393, 4.3) radius 0.5
  circle A3 centre (7.5142, 4.3) radius 0.5
  dimension "d332" = 1
  dimension "d333" = 1
  dimension "d334" = 1
  dimension "d335" = 1
  measures "d332" diameter of A0
  measures "d333" diameter of A1
  measures "d334" diameter of A2
  measures "d335" diameter of A3
extrude "Extrude81" add sketch "Sketch70" along normal blind 2.54 contours A0 | A1 | A2 | A3 bodies 13
sketch "Sketch71" plane through (0, 0, 3) normal (0, 0, 1) x (-1, 0, 0)
  line L0 (9.5, 127.5) -> (9.5, 125)
  line L1 (9.5, 125) -> (10.16, 125)
  line L2 (10.16, 125) -> (10.16, 145.5)
  line L3 (10.16, 145.5) -> (0, 145.5)
  line L4 (0, 145.5) -> (0, 125)
  line L5 (0, 125) -> (0.5, 125)
  line L6 (0.5, 125) -> (0.5, 127.5)
  line L7 (0.5, 127.5) -> (9.5, 127.5)
  circle A0 centre (7, 142.5) radius 2.5495
  line L8 (8.5, 137.5) -> (8.5, 139)
  line L9 (8.5, 139) -> (9.5, 139)
  line L10 (9.5, 139) -> (9.5, 137.5)
  line L11 (9.5, 137.5) -> (8.5, 137.5)
  line L12 (1, 139) -> (1, 144)
  line L13 (1, 144) -> (3.5, 144)
  line L14 (3.5, 144) -> (3.5, 139)
  line L15 (3.5, 139) -> (1, 139)
  line L16 (5, 137) -> (5, 139.5)
  line L17 (5, 139.5) -> (7.5, 139.5)
  line L18 (7.5, 139.5) -> (7.5, 137)
  line L19 (7.5, 137) -> (5, 137)
  line L20 (1, 133.5) -> (9, 133.5) construction
  line L21 (9, 133.5) -> (9, 136.5) construction
  line L22 (9, 136.5) -> (1, 136.5) construction
  line L23 (1, 136.5) -> (1, 133.5) construction
  dimension "d338" = 2
  dimension "d339" = 0
  text T0 "Step Up (12V)" font "Arial" height 2 align centre top in box 8 x 3 at (1, 133.5) x (1, 0) y (0, 1) spacing 1 kerned
extrude "Extrude82" cut sketch "Sketch71" against normal blind 1 text T0 bodies 13
sketch "Sketch72" plane through (0, 0, 0) normal (0, 0, 1) x (1, 0, 0)
  line L0 (-30, -125) -> (-50, -125)
  line L1 (-50, -125) -> (-50, -145)
  line L2 (-50, -145) -> (-30, -145)
  line L3 (-30, -145) -> (-30, -125)
  dimension "d342" = 20
  dimension "d343" = 20
  constraint horizontal L0
  constraint vertical L1
  constraint horizontal L2
  constraint vertical L3
  measures "d342" distance of L0.start L0.end
  measures "d343" distance of L0.start L2.end
extrude "Extrude83" add sketch "Sketch72" along normal blind 3 separate body makes body 14
sketch "Sketch73" plane through (0, 0, 3) normal (0, 0, 1) x (-1, 0, 0)
  line L0 (30, 145) -> (30, 125)
  line L1 (30, 125) -> (50, 125)
  line L2 (50, 125) -> (50, 145)
  line L3 (50, 145) -> (30, 145)
  line L4 (36, 141) -> (44, 141)
  line L5 (44, 141) -> (44, 134)
  line L6 (44, 134) -> (36, 134)
  line L7 (36, 134) -> (36, 141)
  constraint horizontal L4
  constraint vertical L5
  constraint horizontal L6
  constraint vertical L7
extrude "Extrude84" add sketch "Sketch73" along normal blind 1 contours L4 L5 L6 L7 bodies 14
sketch "Sketch74" plane through (0, 0, 3) normal (0, 0, 1) x (-1, 0, 0)
  line L0 (36, 134) -> (36, 141)
  line L1 (36, 141) -> (44, 141)
  line L2 (44, 141) -> (44, 134)
  line L3 (44, 134) -> (36, 134)
  line L4 (30, 145) -> (30, 125)
  line L5 (30, 125) -> (50, 125)
  line L6 (50, 125) -> (50, 145)
  line L7 (50, 145) -> (30, 145)
  line L8 (30.5, 144.5) -> (32.5, 144.5)
  line L9 (32.5, 144.5) -> (32.5, 125.5)
  line L10 (32.5, 125.5) -> (30.5, 125.5)
  line L11 (30.5, 125.5) -> (30.5, 144.5)
  line L12 (49.5, 144.5) -> (47.5, 144.5)
  line L13 (47.5, 144.5) -> (47.5, 125.5)
  line L14 (47.5, 125.5) -> (49.5, 125.5)
  line L15 (49.5, 125.5) -> (49.5, 144.5)
  constraint horizontal L8
  constraint vertical L9
  constraint horizontal L10
  constraint vertical L11
  constraint horizontal L12
  constraint vertical L13
  constraint horizontal L14
  constraint vertical L15
extrude "Extrude85" add sketch "Sketch74" along normal blind 7 contours L8 L9 L10 L11 | L12 L13 L14 L15 bodies 14
sketch "Sketch75" plane through (0, 0, 3) normal (0, 0, 1) x (-1, 0, 0)
  line L0 (49.5, 125.5) -> (47.5, 125.5)
  line L1 (47.5, 125.5) -> (47.5, 144.5)
  line L2 (47.5, 144.5) -> (49.5, 144.5)
  line L3 (49.5, 144.5) -> (49.5, 125.5)
  line L4 (30.5, 125.5) -> (30.5, 144.5)
  line L5 (30.5, 144.5) -> (32.5, 144.5)
  line L6 (32.5, 144.5) -> (32.5, 125.5)
  line L7 (32.5, 125.5) -> (30.5, 125.5)
  line L8 (36, 134) -> (36, 141)
  line L9 (36, 141) -> (44, 141)
  line L10 (44, 141) -> (44, 134)
  line L11 (44, 134) -> (36, 134)
  line L12 (30, 145) -> (30, 125)
  line L13 (30, 125) -> (50, 125)
  line L14 (50, 125) -> (50, 145)
  line L15 (50, 145) -> (30, 145)
  line L16 (35, 130) -> (45, 130) construction
  line L17 (45, 130) -> (45, 132.5) construction
  line L18 (45, 132.5) -> (35, 132.5) construction
  line L19 (35, 132.5) -> (35, 130) construction
  dimension "d350" = 2
  text T0 "MOTOR DRIVER" font "Arial" height 2 align left top in box 10 x 2.5 at (35, 130) x (1, 0) y (0, 1) spacing 1 kerned
extrude "Extrude86" cut sketch "Sketch75" against normal blind 1 text T0 bodies 14
hidden bodies 1
equation "d91 = 'MINI HDMI'"
equation "d93 = 'USB'"
equation "d95 = 'PWR IN'"
equation "d162 = ( 0.83 * 2 ) * 1 mm"
equation "d163 = ( 0.83 * 2 ) * 1 mm"
equation "d164 = ( 0.83 * 2 ) * 1 mm"
equation "d165 = ( 0.83 * 2 ) * 1 mm"
equation "d196 = 'ESP32'"
equation "d200 = 'Pi'"
equation "d204 = 'Pixy2'"
equation "d208 = 'Delta fan'"
equation "d266 = 'ToF'"
equation "d297 = 'IMU'"
equation "d309 = 'Step Down'"
equation "d311 = '(5V)'"
equation "d321 = 'LiPo Battery'"
equation "d339 = 'Step Up (12V)'"
equation "d351 = 'MOTOR DRIVER'"
named bodies: "ANTi sample", "Raspberry Pi Zero 2W", "Pixy 2 Camera", "Arduino Nano ESP32", "Delta fan", "N20 Motor", "ToF #1", "ToF #2", "Servo Motor", "IMU", "Step Down Converter (to 5V)", "LiPo Battery", "Step Up Converter (to 12V)", "Motor Driver"
